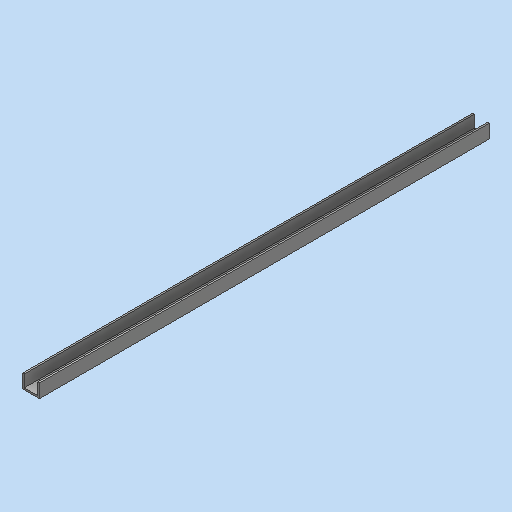
# Autodesk Inventor part: U-Profil PanelSupport 10x8x265mm
Saved by Autodesk Inventor 2023.2 (Build 272271000, 271)
## iProperties
Created: 2023-12-14
Part Number: U-Profil PanelSupport 10x8x265mm
Material: Generisch
Document SubType Name: Modeling
Designer: Nils Bade
Density: 1 g/cm^3
Appearance: Elox-Alu
Description: Nicht vorbestellen, bauhaus
Auf Bestellliste: True
Listed: False
Author: Nils Bade
Autodesk Inventor part; units mm, degrees
ref_plane "YZ Plane" through (0, 0, 0) normal (1, 0, 0) x (0, 1, 0)
ref_plane "XY Plane" through (0, 0, 0) normal (0, 0, 1) x (1, 0, 0)
sketch "Skizze1" plane through (0, 0, 0) normal (0, 0, 1) x (1, 0, 0)
  line L0 (0, 0) -> (5, 0)
  line L1 (5, 0) -> (5, 8)
  line L2 (5, 8) -> (4, 8)
  line L3 (4, 8) -> (4, 1)
  line L4 (4, 1) -> (0, 1)
  line L5 (0, 9.6) -> (0, -1.6) construction
  line L6 (0, 0) -> (-5, 0)
  line L7 (-5, 0) -> (-5, 8)
  line L8 (-5, 8) -> (-4, 8)
  line L9 (-4, 8) -> (-4, 1)
  line L10 (-4, 1) -> (0, 1)
  dimension "d0" = 1
  dimension "d1" = 1
  dimension "d2" = 8
  dimension "d3" = 5
  constraints: 20 end point, 4 perpendicular, 4 symmetric about line, 1 horizontal
  measures "d0" distance between parallel lines of L0 L4
  measures "d1" distance between parallel lines of L3 L1
  measures "d2" distance between parallel lines of L0 L2
  measures "d3" distance of L0.start L0.end
extrude "Ex-UProfil" add sketch "Skizze1" along normal blind 265
sketch "Skizze2" plane through (0, 0, 0) normal (0, 1, 0) x (-1, 0, 0)
  line L0 (5, 0) -> (-5, 0) projected
  line L1 (-5, 0) -> (-5, 265) projected
  line L2 (5, 265) -> (-5, 265) projected
  line L3 (5, 0) -> (5, 265) projected
  line L4 (0, -65.78) -> (0, 302.63) construction
  circle A0 centre (0, 245) radius 2.15 construction
  line L5 (0, 246) -> (0, 244) construction
  line L6 (-2.15, 246) -> (-2.15, 244)
  line L7 (2.15, 244) -> (2.15, 246)
  arc A1 (2.15, 246) -> (-2.15, 246) centre (0, 246) ccw
  arc A2 (-2.15, 244) -> (2.15, 244) centre (0, 244) ccw
  circle A3 centre (0, 165) radius 2.15 construction
  line L8 (0, 166) -> (0, 164) construction
  line L9 (-2.15, 166) -> (-2.15, 164)
  line L10 (2.15, 164) -> (2.15, 166)
  arc A4 (2.15, 166) -> (-2.15, 166) centre (0, 166) ccw
  arc A5 (-2.15, 164) -> (2.15, 164) centre (0, 164) ccw
  circle A6 centre (0, 85) radius 2.15 construction
  line L11 (0, 86) -> (0, 84) construction
  line L12 (-2.15, 86) -> (-2.15, 84)
  line L13 (2.15, 84) -> (2.15, 86)
  arc A7 (2.15, 86) -> (-2.15, 86) centre (0, 86) ccw
  arc A8 (-2.15, 84) -> (2.15, 84) centre (0, 84) ccw
  circle A9 centre (0, 5) radius 2.15 construction
  line L14 (0, 6) -> (0, 4) construction
  line L15 (-2.15, 6) -> (-2.15, 4)
  line L16 (2.15, 4) -> (2.15, 6)
  arc A10 (2.15, 6) -> (-2.15, 6) centre (0, 6) ccw
  arc A11 (-2.15, 4) -> (2.15, 4) centre (0, 4) ccw
  point P0 (0, 0)
  point P1 (0, 248.15)
  point P2 (0, 241.85)
  point P3 (0, 168.15)
  point P4 (0, 161.85)
  point P5 (0, 88.15)
  point P6 (0, 81.85)
  point P7 (0, 8.15)
  point P8 (0, 1.85)
  dimension "d6" = 4.3
  dimension "d7" = 20
  dimension "d8" = 4.3
  dimension "d9" = 6.3
  dimension "d21" = 80
  constraints: 32 end point, 18 point on circle, 12 centre point, 4 tangent, 2 point on line, 1 midpoint, 1 parallel, 1 vertical, 45 other
  measures "d6" diameter of A0
  measures "d7" distance from line of L2 A0.centre
  measures "d8" diameter of A2
  measures "d9" distance of point (0, 248.15) point (0, 241.85)
  measures "d21" distance of A0.centre A3.centre
extrude "Ex-Bohrungen" cut sketch "Skizze2" along normal up to surface (1 mm away) contours A1 L7 A2 L6 | A4 L10 A5 L9 | A7 L13 A8 L12 | A10 L16 A11 L15
equation "\"d8\" = d6"
